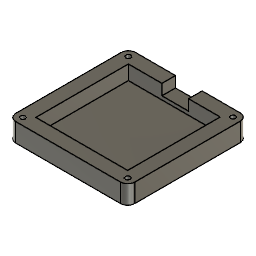
SpeedrunDeck+bottom (Autodesk Fusion 360 archive; units mm, degrees)
design "SpeedrunDeck bottom"
part number: 2025-12-30-21-32-48-708
Autodesk Fusion 360 part; units mm, degrees
sketch "Skectch1" plane through (0, 0, 0) normal (0, 0, 1) x (1, 0, 0)
  line L0 (0, 0) -> (63.9, 0)
  line L1 (63.9, 0) -> (63.9, 64.4)
  line L2 (63.9, 64.4) -> (0, 64.4)
  line L3 (0, 64.4) -> (0, 0)
  line L4 (-9.5, 73.9) -> (73.4, 73.9)
  line L5 (73.4, 73.9) -> (73.4, -9.5)
  line L6 (73.4, -9.5) -> (-9.5, -9.5)
  line L7 (-9.5, -9.5) -> (-9.5, 73.9)
  circle A0 centre (-4.5, -4.5) radius 1.7
  circle A1 centre (68.4, -4.5) radius 1.7
  circle A2 centre (68.4, 68.9) radius 1.7
  circle A3 centre (-4.5, 68.9) radius 1.7
  circle A4 centre (-4.5, -4.5) radius 3
  circle A5 centre (68.4, -4.5) radius 3
  circle A6 centre (68.4, 68.9) radius 3
  circle A7 centre (-4.5, 68.9) radius 3
  dimension "d1" = 63.9
  dimension "d2" = 64.4
  dimension "d3" = 82.9
  dimension "d4" = 83.4
  dimension "d6" = 9.5
  dimension "d7" = 3.4
  dimension "d8" = 5
  dimension "d9" = 5
  dimension "d10" = 3.4
  dimension "d11" = 5
  dimension "d12" = 5
  dimension "d13" = 3.4
  dimension "d14" = 5
  dimension "d15" = 5
  dimension "d16" = 9.5
  dimension "d17" = 3.4
  dimension "d18" = 5
  dimension "d19" = 5
  dimension "d21" = 6
  dimension "d22" = 6
  dimension "d23" = 6
  dimension "d24" = 6
  constraint horizontal L0
  constraint vertical L1
  constraint horizontal L2
  constraint vertical L3
  constraint coincident L0.start L3.end
  constraint horizontal L4
  constraint vertical L5
  constraint horizontal L6
  constraint vertical L7
  constraint concentric A0 A4
  constraint concentric A1 A5
  constraint concentric A2 A6
  constraint concentric A3 A7
  measures "d1" distance of L1.end L2.end
  measures "d2" distance of L0.end L1.end
  measures "d3" distance of L4.start L4.end
  measures "d4" distance of L4.end L5.end
  measures "d6" distance of L1 L5
  measures "d7" diameter of A0
  measures "d8" distance of L7 A0.centre
  measures "d9" distance of L6 A0.centre
  measures "d10" diameter of A1
  measures "d11" distance of L5 A1.centre
  measures "d12" distance of L6 A1.centre
  measures "d13" diameter of A2
  measures "d14" distance of L5 A2.centre
  measures "d15" distance of L4 A2.centre
  measures "d16" distance of L2 L4
  measures "d17" diameter of A3
  measures "d18" distance of L4 A3.centre
  measures "d19" distance of L7 A3.centre
  measures "d21" diameter of A4
  measures "d22" diameter of A5
  measures "d23" diameter of A6
  measures "d24" diameter of A7
extrude "Extrude1" add sketch "Skectch1" along normal blind 9.9 from surface at 3.1 contours A4 | A5 | A6 | A7 makes body 1 at (70.9599, 70.4643, 9.7) makes body 2 at (-1.6809, 67.8739, 9.7) makes body 3 at (69.2125, -1.6121, 9.7) makes body 4 at (-1.5037, -4.6495, 9.7)
extrude "Extrude2" add sketch "Skectch1" along normal blind 13 contours L4 L5 L6 L7 bodies 1 2 3 4
extrude "Extrude3" add sketch "Skectch1" along normal blind 3 contours L0 L1 L2 L3 bodies 1
sketch "Sketch3" plane through (0, 0, 13) normal (0, 0, 1) x (-1, 0, 0)
  circle A0 centre (-68.4, -68.9) radius 1.7
  circle A1 centre (4.5, 4.5) radius 1.7
  line L0 (0, 0) -> (0, -64.4)
  line L1 (0, -64.4) -> (-63.9, -64.4)
  line L2 (-63.9, -64.4) -> (-63.9, 0)
  line L3 (-63.9, 0) -> (0, 0)
  line L4 (9.5, 9.5) -> (-73.4, 9.5)
  line L5 (-73.4, 9.5) -> (-73.4, -73.9)
  line L6 (-73.4, -73.9) -> (9.5, -73.9)
  line L7 (9.5, -73.9) -> (9.5, 9.5)
  circle A2 centre (4.5, -68.9) radius 1.7
  circle A3 centre (-68.4, 4.5) radius 1.7
  line L8 (-23.35, -73.9) -> (-41.85, -73.9)
  line L9 (-41.85, -73.9) -> (-41.85, -64.4)
  line L10 (-41.85, -64.4) -> (-23.35, -64.4)
  line L11 (-23.35, -64.4) -> (-23.35, -73.9)
  line L12 (9.5, 9.5) -> (9.5, -73.9)
  line L13 (-73.4, -73.9) -> (-73.4, 9.5)
  dimension "d32" = 18.5
  dimension "d33" = 32.85
  dimension "d34" = 31.55
  constraint horizontal L8
  constraint vertical L9
  constraint horizontal L10
  constraint vertical L11
  constraint coincident L1 L9.end
  constraint coincident L6 L8.start
  measures "d32" distance of L8.start L8.end
  measures "d33" distance of L11 L12
  measures "d34" distance of L9 L13
extrude "Extrude4" cut sketch "Sketch3" against normal blind 7.5 contours L1 L6 L8 L9 L10 L11 bodies 1
fillet "Fillet1" radius 5 4 edges at (73.4, -9.5, 6.5) (73.4, 73.9, 6.5) (-9.5, 73.9, 6.5) (-9.5, -9.5, 6.5) on bodies 1
